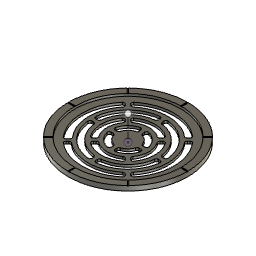
Banc de test part 2 (Autodesk Fusion 360 design; units mm, degrees)
Autodesk Fusion 360 part; units mm, degrees
sketch "Esquisse1" plane through (0, 0, 0) normal (0, 0, 1) x (1, 0, 0)
  circle A0 centre (0, 0) radius 62.5
  dimension "d1" = 125
  constraint coincident A0.centre origin
  measures "d1" diameter of A0
extrude "Extrusion1" add sketch "Esquisse1" along normal blind 5
sketch "Esquisse2" plane through (0, 0, 5) normal (0, 0, 1) x (-1, 0, 0)
  circle A0 centre (0, 0) radius 62.5
  circle A1 centre (0, 0) radius 55.5
  dimension "d4" = 111
  constraint coincident A0.centre A1.centre
  measures "d4" diameter of A1
extrude "Extrusion2" cut sketch "Esquisse2" against normal blind 2.5 contours A1
sketch "Esquisse4" plane through (0, 0, 0) normal (1, 0, 0) x (0, 1, 0)
  line L0 (0, 0) -> (0, 26) construction
  constraint coincident L0.start origin
  constraint vertical L0
sketch "Esquisse3" plane through (0, 0, 5) normal (0, 0, 1) x (-1, 0, 0)
  circle A0 centre (0, 0) radius 55.5
  circle A1 centre (0, 0) radius 62.5
  line L0 (0.5411, -55.4974) -> (0.5411, -62.4977)
  line L1 (-0.4589, -62.4983) -> (-0.4589, -55.4981)
  line L2 (43.8684, -44.5176) -> (38.6533, -39.3025)
  line L3 (39.3599, -38.5949) -> (44.575, -43.81)
  line L4 (62.4983, -0.459) -> (55.1231, -0.459)
  line L5 (55.1223, 0.541) -> (62.4977, 0.541)
  line L6 (44.5176, 43.8684) -> (39.3025, 38.6533)
  line L7 (38.5949, 39.3599) -> (43.81, 44.575)
  line L8 (0.459, 62.4983) -> (0.459, 55.1231)
  line L9 (-0.541, 55.1223) -> (-0.541, 62.4977)
  line L10 (-43.8684, 44.5176) -> (-38.6533, 39.3025)
  line L11 (-39.3599, 38.5949) -> (-44.575, 43.81)
  line L12 (-62.4983, 0.459) -> (-55.1231, 0.459)
  line L13 (-55.1223, -0.541) -> (-62.4977, -0.541)
  line L14 (-38.5949, -39.3599) -> (-43.81, -44.575)
  line L15 (-44.5176, -43.8684) -> (-39.3025, -38.6533)
  dimension "d7" = 1
  dimension "d8" = 1
  dimension "d9" = 1
  dimension "d10" = 1
  dimension "d11" = 1
  dimension "d12" = 1
  dimension "d13" = 1
  dimension "d14" = 1
  constraint coincident A0 L0.start
  constraint coincident A1 L0.end
  constraint vertical L0
  constraint coincident A1 L1.start
  constraint coincident A0 L1.end
  constraint parallel L0 L1
  constraint parallel L2 L3
  constraint parallel L4 L5
  constraint parallel L6 L7
  constraint parallel L8 L9
  constraint parallel L10 L11
  constraint parallel L12 L13
  constraint parallel L14 L15
  measures "d7" distance of L0 L1
  measures "d8" distance of L2 L3
  measures "d9" distance of L4 L5
  measures "d10" distance of L6 L7
  measures "d11" distance of L8 L9
  measures "d12" distance of L10 L11
  measures "d13" distance of L12 L13
  measures "d14" distance of L14 L15
extrude "Extrusion3" cut sketch "Esquisse3" against normal blind 0.5 contours A0 A1 L0 L1 | A0 A1 L14 L15 | A0 A1 L2 L3 | A0 A1 L12 L13 | A0 A1 L4 L5 | A0 A1 L10 L11 | A0 A1 L6 L7 | A0 A1 L8 L9
sketch "Esquisse5" plane through (0, 0, 2.5) normal (0, 0, 1) x (-1, 0, 0)
  circle A0 centre (0, 0) radius 55.5
  line L0 (-2, -15.4919) -> (-2, -13.4164)
  arc A1 (-11.4998, -3.4286) -> (-3.4286, -11.4998) centre (0, 0) ccw
  line L1 (-15.4919, -2) -> (-13.4164, -2)
  arc A2 (-17.4284, -4.5) -> (-4.5, -17.4284) centre (0, 0) ccw
  arc A3 (-3.4286, 11.4998) -> (-11.4998, 3.4286) centre (0, 0) ccw
  line L2 (-15.4919, 2) -> (-13.4164, 2)
  arc A4 (-4.5, 17.4284) -> (-17.4284, 4.5) centre (0, 0) ccw
  line L3 (-2, 13.4164) -> (-2, 15.4919)
  arc A5 (11.4998, 3.4286) -> (3.4286, 11.4998) centre (0, 0) ccw
  line L4 (2, 13.4164) -> (2, 15.4919)
  arc A6 (17.4284, 4.5) -> (4.5, 17.4284) centre (0, 0) ccw
  line L5 (15.4919, 2) -> (13.4164, 2)
  line L6 (15.4919, -2) -> (13.4164, -2)
  arc A7 (2.7692, -11.6761) -> (11.4998, -3.4286) centre (0, 0) ccw
  line L7 (2, -15.4919) -> (2, -12.6491)
  arc A8 (4.5, -17.4284) -> (17.4284, -4.5) centre (0, 0) ccw
  arc A9 (-17.9315, 12.746) -> (-17.9315, -12.746) centre (0, 0) ccw
  line L8 (-18.1474, -15.319) -> (-19.5801, -16.7517)
  arc A10 (-22.6093, 16.5173) -> (-22.6093, -16.5173) centre (0, 0) ccw
  line L9 (-18.1474, 15.319) -> (-19.5801, 16.7517)
  line L10 (-15.319, -18.1474) -> (-16.7517, -19.5801)
  arc A11 (-16.5173, -22.6093) -> (16.5173, -22.6093) centre (0, 0) ccw
  line L11 (15.319, -18.1474) -> (16.7517, -19.5801)
  arc A12 (-12.746, -17.9315) -> (12.746, -17.9315) centre (0, 0) ccw
  line L12 (18.1474, -15.319) -> (19.5801, -16.7517)
  arc A13 (22.6093, -16.5173) -> (22.6093, 16.5173) centre (0, 0) ccw
  line L13 (18.1474, 15.319) -> (19.5801, 16.7517)
  arc A14 (17.9315, -12.746) -> (17.9315, 12.746) centre (0, 0) ccw
  line L14 (15.319, 18.1474) -> (16.7517, 19.5801)
  arc A15 (16.5173, 22.6093) -> (-16.5173, 22.6093) centre (0, 0) ccw
  line L15 (-15.319, 18.1474) -> (-16.7517, 19.5801)
  arc A16 (12.746, 17.9315) -> (-12.746, 17.9315) centre (0, 0) ccw
  line L16 (33.7639, 2) -> (35.7771, 2)
  arc A17 (37.7647, 4.2222) -> (4.2222, 37.7647) centre (0, 0) ccw
  line L17 (2, 33.7639) -> (2, 35.7771)
  arc A18 (31.7778, 3.7647) -> (3.7647, 31.7778) centre (0, 0) ccw
  line L18 (33.7639, -2) -> (35.7771, -2)
  arc A19 (4.2222, -37.7647) -> (37.7647, -4.2222) centre (0, 0) ccw
  line L19 (2, -33.7639) -> (2, -35.7771)
  arc A20 (3.7647, -31.7778) -> (31.7778, -3.7647) centre (0, 0) ccw
  line L20 (29.5697, 32.3981) -> (30.9895, 33.8179)
  arc A21 (30.8612, 36.764) -> (-30.8612, 36.764) centre (0, 0) ccw
  line L21 (-29.5697, 32.3981) -> (-30.9895, 33.8179)
  arc A22 (26.8756, 32.2754) -> (-26.8756, 32.2754) centre (0, 0) ccw
  line L22 (31.1586, 29.6028) -> (33.1753, 31.6675)
  arc A23 (36.7645, -30.8601) -> (36.1114, 31.5869) centre (-0.0189, -0.0179) ccw
  line L23 (32.3901, -29.5617) -> (33.8177, -30.9893)
  arc A24 (32.2502, -26.8887) -> (31.0909, 26.8807) centre (-0.097, -0.6889) ccw
  line L24 (29.5697, -32.3981) -> (30.9895, -33.8179)
  arc A25 (-30.8612, -36.764) -> (30.8612, -36.764) centre (0, 0) ccw
  line L25 (-29.5697, -32.3981) -> (-30.9895, -33.8179)
  arc A26 (-26.8756, -32.2754) -> (26.8756, -32.2754) centre (0, 0) ccw
  line L26 (-2, -33.7639) -> (-2, -35.7771)
  arc A27 (-37.7647, -4.2222) -> (-4.2222, -37.7647) centre (0, 0) ccw
  line L27 (-33.7639, -2) -> (-35.7771, -2)
  arc A28 (-31.7778, -3.7647) -> (-3.7647, -31.7778) centre (0, 0) ccw
  line L28 (-33.7639, 2) -> (-35.7771, 2)
  arc A29 (-4.2222, 37.7647) -> (-37.7647, 4.2222) centre (0, 0) ccw
  line L29 (-2, 33.7639) -> (-2, 35.7771)
  arc A30 (-3.7647, 31.7778) -> (-31.7778, 3.7647) centre (0, 0) ccw
  line L30 (-32.3981, 29.5697) -> (-33.8179, 30.9895)
  arc A31 (-36.764, 30.8612) -> (-36.764, -30.8612) centre (0, 0) ccw
  line L31 (-32.3981, -29.5697) -> (-33.8179, -30.9895)
  arc A32 (-32.2754, 26.8756) -> (-32.2754, -26.8756) centre (0, 0) ccw
  arc A33 (36.1114, 31.5869) -> (33.1753, 31.6675) centre (34.6061, 30.2701) ccw
  arc A34 (31.1586, 29.6028) -> (31.0909, 26.8807) centre (32.5894, 28.2053) ccw
  arc A35 (33.8177, -30.9893) -> (36.7645, -30.8601) centre (35.232, -29.5751) ccw
  arc A36 (32.2502, -26.8887) -> (32.3901, -29.5617) centre (33.8043, -28.1475) ccw
  arc A37 (30.9895, 33.8179) -> (30.8612, 36.764) centre (29.5753, 35.2321) ccw
  arc A38 (26.8756, 32.2754) -> (29.5697, 32.3981) centre (28.1554, 33.8123) ccw
  arc A39 (-29.5697, 32.3981) -> (-26.8756, 32.2754) centre (-28.1554, 33.8123) ccw
  arc A40 (-30.8612, 36.764) -> (-30.9895, 33.8179) centre (-29.5753, 35.2321) ccw
  arc A41 (-33.8179, 30.9895) -> (-36.764, 30.8612) centre (-35.2321, 29.5753) ccw
  arc A42 (-32.2754, 26.8756) -> (-32.3981, 29.5697) centre (-33.8123, 28.1554) ccw
  arc A43 (-36.764, -30.8612) -> (-33.8179, -30.9895) centre (-35.2321, -29.5753) ccw
  arc A44 (-32.3981, -29.5697) -> (-32.2754, -26.8756) centre (-33.8123, -28.1554) ccw
  arc A45 (-30.9895, -33.8179) -> (-30.8612, -36.764) centre (-29.5753, -35.2321) ccw
  arc A46 (-26.8756, -32.2754) -> (-29.5697, -32.3981) centre (-28.1554, -33.8123) ccw
  arc A47 (30.8612, -36.764) -> (30.9895, -33.8179) centre (29.5753, -35.2321) ccw
  arc A48 (29.5697, -32.3981) -> (26.8756, -32.2754) centre (28.1554, -33.8123) ccw
  arc A49 (37.7647, -4.2222) -> (35.7771, -2) centre (35.7771, -4) ccw
  arc A50 (35.7771, 2) -> (37.7647, 4.2222) centre (35.7771, 4) ccw
  arc A51 (33.7639, -2) -> (31.7778, -3.7647) centre (33.7639, -4) ccw
  arc A52 (31.7778, 3.7647) -> (33.7639, 2) centre (33.7639, 4) ccw
  arc A53 (2, -35.7771) -> (4.2222, -37.7647) centre (4, -35.7771) ccw
  arc A54 (-4.2222, -37.7647) -> (-2, -35.7771) centre (-4, -35.7771) ccw
  arc A55 (-2, -33.7639) -> (-3.7647, -31.7778) centre (-4, -33.7639) ccw
  arc A56 (3.7647, -31.7778) -> (2, -33.7639) centre (4, -33.7639) ccw
  arc A57 (4.2222, 37.7647) -> (2, 35.7771) centre (4, 35.7771) ccw
  arc A58 (-2, 35.7771) -> (-4.2222, 37.7647) centre (-4, 35.7771) ccw
  arc A59 (2, 33.7639) -> (3.7647, 31.7778) centre (4, 33.7639) ccw
  arc A60 (-3.7647, 31.7778) -> (-2, 33.7639) centre (-4, 33.7639) ccw
  arc A61 (-37.7647, 4.2222) -> (-35.7771, 2) centre (-35.7771, 4) ccw
  arc A62 (-33.7639, 2) -> (-31.7778, 3.7647) centre (-33.7639, 4) ccw
  arc A63 (-31.7778, -3.7647) -> (-33.7639, -2) centre (-33.7639, -4) ccw
  arc A64 (-35.7771, -2) -> (-37.7647, -4.2222) centre (-35.7771, -4) ccw
  arc A65 (-17.9315, 12.746) -> (-18.1474, 15.319) centre (-19.5616, 13.9048) ccw
  arc A66 (-15.319, 18.1474) -> (-12.746, 17.9315) centre (-13.9048, 19.5616) ccw
  arc A67 (12.746, 17.9315) -> (15.319, 18.1474) centre (13.9048, 19.5616) ccw
  arc A68 (-18.1474, -15.319) -> (-17.9315, -12.746) centre (-19.5616, -13.9048) ccw
  arc A69 (-12.746, -17.9315) -> (-15.319, -18.1474) centre (-13.9048, -19.5616) ccw
  arc A70 (18.1474, 15.319) -> (17.9315, 12.746) centre (19.5616, 13.9048) ccw
  arc A71 (-16.5173, 22.6093) -> (-16.7517, 19.5801) centre (-15.3375, 20.9943) ccw
  arc A72 (-19.5801, 16.7517) -> (-22.6093, 16.5173) centre (-20.9943, 15.3375) ccw
  arc A73 (-22.6093, -16.5173) -> (-19.5801, -16.7517) centre (-20.9943, -15.3375) ccw
  arc A74 (-16.7517, -19.5801) -> (-16.5173, -22.6093) centre (-15.3375, -20.9943) ccw
  arc A75 (16.7517, 19.5801) -> (16.5173, 22.6093) centre (15.3375, 20.9943) ccw
  arc A76 (22.6093, 16.5173) -> (19.5801, 16.7517) centre (20.9943, 15.3375) ccw
  arc A77 (17.9315, -12.746) -> (18.1474, -15.319) centre (19.5616, -13.9048) ccw
  arc A78 (15.319, -18.1474) -> (12.746, -17.9315) centre (13.9048, -19.5616) ccw
  arc A79 (16.5173, -22.6093) -> (16.7517, -19.5801) centre (15.3375, -20.9943) ccw
  arc A80 (19.5801, -16.7517) -> (22.6093, -16.5173) centre (20.9943, -15.3375) ccw
  arc A81 (17.4284, -4.5) -> (15.4919, -2) centre (15.4919, -4) ccw
  arc A82 (15.4919, 2) -> (17.4284, 4.5) centre (15.4919, 4) ccw
  arc A83 (4.5, 17.4284) -> (2, 15.4919) centre (4, 15.4919) ccw
  arc A84 (-2, 15.4919) -> (-4.5, 17.4284) centre (-4, 15.4919) ccw
  arc A85 (-17.4284, 4.5) -> (-15.4919, 2) centre (-15.4919, 4) ccw
  arc A86 (-15.4919, -2) -> (-17.4284, -4.5) centre (-15.4919, -4) ccw
  arc A87 (-4.5, -17.4284) -> (-2, -15.4919) centre (-4, -15.4919) ccw
  arc A88 (2, -15.4919) -> (4.5, -17.4284) centre (4, -15.4919) ccw
  arc A89 (13.4164, -2) -> (11.4998, -3.4286) centre (13.4164, -4) ccw
  arc A90 (2.7692, -11.6761) -> (2, -12.6491) centre (3, -12.6491) ccw
  arc A91 (-2, -13.4164) -> (-3.4286, -11.4998) centre (-4, -13.4164) ccw
  arc A92 (-11.4998, -3.4286) -> (-13.4164, -2) centre (-13.4164, -4) ccw
  arc A93 (-13.4164, 2) -> (-11.4998, 3.4286) centre (-13.4164, 4) ccw
  arc A94 (-3.4286, 11.4998) -> (-2, 13.4164) centre (-4, 13.4164) ccw
  arc A95 (2, 13.4164) -> (3.4286, 11.4998) centre (4, 13.4164) ccw
  arc A96 (11.4998, 3.4286) -> (13.4164, 2) centre (13.4164, 4) ccw
  dimension "d38" = 2
  dimension "d39" = 2
  dimension "d40" = 2
  dimension "d41" = 2
  dimension "d42" = 2
  dimension "d43" = 2
  dimension "d44" = 2
  dimension "d45" = 2
  dimension "d46" = 2
  dimension "d47" = 2
  dimension "d48" = 2
  dimension "d49" = 2
  dimension "d50" = 2
  dimension "d51" = 2
  dimension "d52" = 2
  dimension "d53" = 2
  dimension "d54" = 2
  dimension "d55" = 2
  dimension "d56" = 2
  dimension "d57" = 2
  dimension "d58" = 2
  dimension "d59" = 2
  dimension "d60" = 2
  dimension "d61" = 2
  dimension "d62" = 2
  dimension "d63" = 2
  dimension "d64" = 2
  dimension "d65" = 2
  dimension "d66" = 2
  dimension "d67" = 2
  dimension "d68" = 2
  dimension "d69" = 2
  dimension "d70" = 2
  dimension "d71" = 2
  dimension "d72" = 2
  dimension "d73" = 2
  dimension "d74" = 2
  dimension "d75" = 2
  dimension "d76" = 2
  dimension "d77" = 2
  dimension "d78" = 2
  dimension "d79" = 2
  dimension "d80" = 2
  dimension "d81" = 2
  dimension "d82" = 2
  dimension "d83" = 2
  dimension "d84" = 2
  dimension "d85" = 2
  dimension "d86" = 2
  dimension "d87" = 2
  dimension "d88" = 2
  dimension "d89" = 2
  dimension "d90" = 2
  dimension "d91" = 2
  dimension "d92" = 2
  dimension "d93" = 2
  dimension "d94" = 2
  dimension "d95" = 1
  dimension "d96" = 2
  dimension "d97" = 2
  dimension "d98" = 2
  dimension "d99" = 2
  dimension "d100" = 2
  dimension "d101" = 2
  constraint tangent A23 A33
  constraint tangent L22 A33
  constraint tangent L22 A34
  constraint tangent A24 A34
  constraint tangent A23 A35
  constraint tangent L23 A35
  constraint tangent A24 A36
  constraint tangent L23 A36
  constraint tangent A21 A37
  constraint tangent L20 A37
  constraint tangent A22 A38
  constraint tangent L20 A38
  constraint tangent A22 A39
  constraint tangent L21 A39
  constraint tangent L21 A40
  constraint tangent A21 A40
  constraint tangent A31 A41
  constraint tangent L30 A41
  constraint tangent A32 A42
  constraint tangent L30 A42
  constraint tangent A31 A43
  constraint tangent L31 A43
  constraint tangent L31 A44
  constraint tangent A32 A44
  constraint tangent A25 A45
  constraint tangent L25 A45
  constraint tangent L25 A46
  constraint tangent A26 A46
  constraint tangent L24 A47
  constraint tangent A25 A47
  constraint tangent L24 A48
  constraint tangent A26 A48
  constraint tangent A19 A49
  constraint tangent L18 A49
  constraint tangent L16 A50
  constraint tangent A17 A50
  constraint tangent L18 A51
  constraint tangent A20 A51
  constraint tangent A18 A52
  constraint tangent L16 A52
  constraint tangent A19 A53
  constraint tangent L19 A53
  constraint tangent L26 A54
  constraint tangent A27 A54
  constraint tangent L26 A55
  constraint tangent A28 A55
  constraint tangent L19 A56
  constraint tangent A20 A56
  constraint tangent A17 A57
  constraint tangent L17 A57
  constraint tangent L29 A58
  constraint tangent A29 A58
  constraint tangent A18 A59
  constraint tangent L17 A59
  constraint tangent L29 A60
  constraint tangent A30 A60
  constraint tangent A29 A61
  constraint tangent L28 A61
  constraint tangent L28 A62
  constraint tangent A30 A62
  constraint tangent L27 A63
  constraint tangent A28 A63
  constraint tangent L27 A64
  constraint tangent A27 A64
  constraint tangent L9 A65
  constraint tangent A9 A65
  constraint tangent A16 A66
  constraint tangent L15 A66
  constraint tangent A16 A67
  constraint tangent L14 A67
  constraint tangent A9 A68
  constraint tangent L8 A68
  constraint tangent A12 A69
  constraint tangent L10 A69
  constraint tangent A14 A70
  constraint tangent L13 A70
  constraint tangent L15 A71
  constraint tangent A15 A71
  constraint tangent L9 A72
  constraint tangent A10 A72
  constraint tangent A10 A73
  constraint tangent L8 A73
  constraint tangent A11 A74
  constraint tangent L10 A74
  constraint tangent A15 A75
  constraint tangent L14 A75
  constraint tangent L13 A76
  constraint tangent A13 A76
  constraint tangent L12 A77
  constraint tangent A14 A77
  constraint tangent L11 A78
  constraint tangent A12 A78
  constraint tangent A11 A79
  constraint tangent L11 A79
  constraint tangent L12 A80
  constraint tangent A13 A80
  constraint tangent A8 A81
  constraint tangent L6 A81
  constraint tangent L5 A82
  constraint tangent A6 A82
  constraint tangent A6 A83
  constraint tangent L4 A83
  constraint tangent L3 A84
  constraint tangent A4 A84
  constraint tangent A4 A85
  constraint tangent L2 A85
  constraint tangent L1 A86
  constraint tangent A2 A86
  constraint tangent A2 A87
  constraint tangent L0 A87
  constraint tangent L7 A88
  constraint tangent A8 A88
  constraint tangent A7 A89
  constraint tangent L6 A89
  constraint tangent L7 A90
  constraint tangent A7 A90
  constraint tangent L0 A91
  constraint tangent A1 A91
  constraint tangent L1 A92
  constraint tangent A1 A92
  constraint tangent L2 A93
  constraint tangent A3 A93
  constraint tangent A3 A94
  constraint tangent L3 A94
  constraint tangent L4 A95
  constraint tangent A5 A95
  constraint tangent A5 A96
  constraint tangent L5 A96
  measures "d38" radius of A33
  measures "d39" radius of A34
  measures "d40" radius of A35
  measures "d41" radius of A36
  measures "d42" radius of A37
  measures "d43" radius of A38
  measures "d44" radius of A39
  measures "d45" radius of A40
  measures "d46" radius of A41
  measures "d47" radius of A42
  measures "d48" radius of A43
  measures "d49" radius of A44
  measures "d50" radius of A45
  measures "d51" radius of A46
  measures "d52" radius of A47
  measures "d53" radius of A48
  measures "d54" radius of A49
  measures "d55" radius of A50
  measures "d56" radius of A51
  measures "d57" radius of A52
  measures "d58" radius of A53
  measures "d59" radius of A54
  measures "d60" radius of A55
  measures "d61" radius of A56
  measures "d62" radius of A57
  measures "d63" radius of A58
  measures "d64" radius of A59
  measures "d65" radius of A60
  measures "d66" radius of A61
  measures "d67" radius of A62
  measures "d68" radius of A63
  measures "d69" radius of A64
  measures "d70" radius of A65
  measures "d71" radius of A66
  measures "d72" radius of A67
  measures "d73" radius of A68
  measures "d74" radius of A69
  measures "d75" radius of A70
  measures "d76" radius of A71
  measures "d77" radius of A72
  measures "d78" radius of A73
  measures "d79" radius of A74
  measures "d80" radius of A75
  measures "d81" radius of A76
  measures "d82" radius of A77
  measures "d83" radius of A78
  measures "d84" radius of A79
  measures "d85" radius of A80
  measures "d86" radius of A81
  measures "d87" radius of A82
  measures "d88" radius of A83
  measures "d89" radius of A84
  measures "d90" radius of A85
  measures "d91" radius of A86
  measures "d92" radius of A87
  measures "d93" radius of A88
  measures "d94" radius of A89
  measures "d95" radius of A90
  measures "d96" radius of A91
  measures "d97" radius of A92
  measures "d98" radius of A93
  measures "d99" radius of A94
  measures "d100" radius of A95
  measures "d101" radius of A96
extrude "Extrusion4" cut sketch "Esquisse5" against normal blind 5 contours L0 A1 L1 A2 A86 A87 A91 A92 | A3 L2 A4 L3 A84 A85 A93 A94 | A5 L4 A6 L5 A82 A83 A95 A96 | L6 A7 L7 A8 A81 A88 A89 A90 | A9 L8 A10 L9 A65 A68 A72 A73 | L10 A11 L11 A12 A69 A74 A78 A79 | L12 A13 L13 A14 A70 A76 A77 A80 | L14 A15 L15 A16 A66 A67 A71 A75 | L16 A17 L17 A18 A50 A52 A57 A59 | L18 A19 L19 A20 A49 A51 A53 A56 | L20 A21 L21 A22 A37 A38 A39 A40 | L22 A23 L23 A24 A33 A34 A35 A36 | L24 A25 L25 A26 A45 A46 A47 A48 | L26 A27 L27 A28 A54 A55 A63 A64 | L28 A29 L29 A30 A58 A60 A61 A62 | L30 A31 L31 A32 A41 A42 A43 A44
